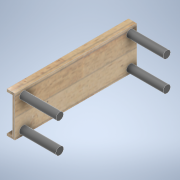
# Autodesk Inventor part: TABLE FOR VERTI
Saved by Autodesk Inventor 2021 (Build 250183000, 183)
## iProperties
Created: 2021-07-15
Part Number: TABLE FOR VERTI
Material: Wood (Maple)
Document SubType Name: Modeling
Designer: HP
Density: 0.67 g/cm^3
Appearance: Natural Maple - Glossy Dark Tint
Author: HP
Autodesk Inventor part; units mm, degrees
ref_plane "YZ Plane" through (0, 0, 0) normal (1, 0, 0) x (0, 1, 0)
ref_plane "XZ Plane" through (0, 0, 0) normal (0, 1, 0) x (-1, 0, 0)
ref_plane "XY Plane" through (0, 0, 0) normal (0, 0, 1) x (1, 0, 0)
sketch "Sketch1" plane through (0, 0, 0) normal (1, 0, 0) x (0, 1, 0)
  line L0 (-76.2, 25.8729) -> (-203.2, 25.8729)
  line L1 (-203.2, 25.8729) -> (-203.2, -355.1271)
  line L2 (-203.2, -355.1271) -> (-76.2, -355.1271)
  line L3 (-76.2, -355.1271) -> (-76.2, 25.8729)
  point P0 (0, 0)
  dimension "d0" = 127
  dimension "d1" = 381
  constraints: 8 end point, 2 parallel, 1 horizontal, 1 perpendicular
  measures "d0" distance of L2.end L1.end
  measures "d1" distance of L1.end L0.end
extrude "Extrusion1" add sketch "Sketch1" along normal blind 7.62
sketch "Sketch2" plane through (7.62, 0, 0) normal (1, 0, 0) x (0, 0, -1)
  circle A0 centre (0, -187.325) radius 11.9854
  circle A1 centre (334.9625, -187.325) radius 11.557
  point P0 (0, 0)
  dimension "d5" = 23.114
  constraints: 2 centre point
  measures "d5" diameter of A1
extrude "Extrusion2" add sketch "Sketch2" along normal blind 114.3
sketch "Sketch3" plane through (7.62, 0, 0) normal (1, 0, 0) x (0, 0, -1)
  circle A0 centre (0, -93.6625) radius 11.557
  circle A1 centre (334.9625, -93.6625) radius 11.557
  point P0 (0, 0)
  dimension "d8" = 23.114
  dimension "d9" = 23.114
  constraints: 2 centre point
  measures "d8" diameter of A0
  measures "d9" diameter of A1
extrude "Extrusion3" add sketch "Sketch3" along normal blind 114.3
sketch "Sketch4" plane through (0, 0, 0) normal (-1, 0, 0) x (0, 0, 1)
  line L0 (25.8729, -76.2) -> (25.8729, -203.2) projected
  line L1 (-355.1271, -203.2) -> (-355.1271, -76.2) projected
  line L2 (25.8729, -203.2) -> (-355.1271, -203.2)
  line L3 (-355.1271, -203.2) -> (-355.1271, -196.85)
  line L4 (-355.1271, -196.85) -> (25.8729, -196.85)
  line L5 (25.8729, -196.85) -> (25.8729, -203.2)
  line L6 (-355.1271, -76.2) -> (25.8729, -76.2) projected
  line L7 (-355.1271, -196.85) -> (-347.1769, -196.85)
  line L8 (-347.1769, -196.85) -> (-347.1769, -76.2)
  line L9 (-347.1769, -76.2) -> (-355.1271, -76.2)
  line L10 (-355.1271, -76.2) -> (-355.1271, -196.85)
  line L11 (25.8729, -84.1375) -> (-355.1271, -84.1375)
  line L12 (-355.1271, -84.1375) -> (-355.1271, -76.2)
  line L13 (-355.1271, -76.2) -> (25.8729, -76.2)
  line L14 (25.8729, -76.2) -> (25.8729, -84.1375)
  point P0 (0, 0)
  point P1 (25.8729, -196.85)
  point P2 (-347.1769, -84.1375)
  dimension "d12" = 7.9502
  constraints: 24 end point, 6 parallel, 3 horizontal, 3 perpendicular, 3 point on line
  measures "d12" distance of L9.end L8.end
extrude "Extrusion4" add sketch "Sketch4" along normal blind 17.78 contours L0 L11 L8 L6 | L8 L11 L1 L6 | L0 L2 L1 L4 | L8 L4 L1 L11
body "Solid1"
